Autodesk Fusion 360 part; units mm, degrees
note: some values were not read from the file. Set by a fixed rule: which sketch regions a step uses.
(part 2 of 2)
sketch "Sketch3" plane through (0, 0, 0) normal (0, 0, -1) x (1, 0, 0)
  line L0 (-14.5833, -10.5) -> (-14.5833, -10.5839)
  arc A0 (-8, -23) -> (-14.5833, -10.5839) centre (-23, -23) ccw
  line L1 (-8, -23) -> (-8, -42.8293)
  arc A1 (-10.0769, -45.2933) -> (-8, -42.8293) centre (-10.5, -42.8293) ccw
  arc A2 (-10.0769, -45.2933) -> (-10.4615, -55.0673) centre (-9.2308, -50.2212) ccw
  arc A3 (-10.4615, -55.0673) -> (10.4615, -55.0673) centre (0, -13.875) ccw
  arc A4 (10.4615, -55.0673) -> (10.0769, -45.2933) centre (9.2308, -50.2212) ccw
  arc A5 (8, -42.8293) -> (10.0769, -45.2933) centre (10.5, -42.8293) ccw
  line L2 (8, -42.8293) -> (8, -23)
  arc A6 (14.5833, -10.5839) -> (8, -23) centre (23, -23) ccw
  line L3 (14.5833, -10.5839) -> (14.5833, -10.5)
  line L4 (14.5833, -10.5) -> (14.7084, -10.5)
  arc A7 (23, -8) -> (14.7084, -10.5) centre (23, -23) ccw
  line L5 (23, -8) -> (42.8293, -8)
  arc A8 (45.2933, -10.0769) -> (42.8293, -8) centre (42.8293, -10.5) ccw
  arc A9 (45.2933, -10.0769) -> (55.0673, -10.4615) centre (50.2212, -9.2308) ccw
  arc A10 (55.0673, -10.4615) -> (55.0673, 10.4615) centre (13.875, 0) ccw
  arc A11 (55.0673, 10.4615) -> (45.2933, 10.0769) centre (50.2212, 9.2308) ccw
  arc A12 (42.8293, 8) -> (45.2933, 10.0769) centre (42.8293, 10.5) ccw
  line L6 (42.8293, 8) -> (23, 8)
  arc A13 (8, 23) -> (23, 8) centre (23, 23) ccw
  line L7 (8, 23) -> (8, 42.8293)
  arc A14 (10.0769, 45.2933) -> (8, 42.8293) centre (10.5, 42.8293) ccw
  arc A15 (10.0769, 45.2933) -> (10.4615, 55.0673) centre (9.2308, 50.2212) ccw
  arc A16 (10.4615, 55.0673) -> (-10.4615, 55.0673) centre (0, 13.875) ccw
  arc A17 (-10.4615, 55.0673) -> (-10.0769, 45.2933) centre (-9.2308, 50.2212) ccw
  arc A18 (-8, 42.8293) -> (-10.0769, 45.2933) centre (-10.5, 42.8293) ccw
  line L8 (-8, 42.8293) -> (-8, 23)
  arc A19 (-23, 8) -> (-8, 23) centre (-23, 23) ccw
  line L9 (-23, 8) -> (-42.8293, 8)
  arc A20 (-45.2933, 10.0769) -> (-42.8293, 8) centre (-42.8293, 10.5) ccw
  arc A21 (-45.2933, 10.0769) -> (-55.0673, 10.4615) centre (-50.2212, 9.2308) ccw
  arc A22 (-55.0673, 10.4615) -> (-55.0673, -10.4615) centre (-13.875, 0) ccw
  arc A23 (-55.0673, -10.4615) -> (-45.2933, -10.0769) centre (-50.2212, -9.2308) ccw
  arc A24 (-42.8293, -8) -> (-45.2933, -10.0769) centre (-42.8293, -10.5) ccw
  line L10 (-42.8293, -8) -> (-23, -8)
  arc A25 (-14.7084, -10.5) -> (-23, -8) centre (-23, -23) ccw
  line L11 (-14.7084, -10.5) -> (-14.5833, -10.5)
  line L12 (-8.3333, -9.25) -> (-8.3333, -5.25)
  line L13 (-8.3333, -5.25) -> (-10.3333, -5.25)
  line L14 (-10.3333, -5.25) -> (-10.3333, -3.25)
  line L15 (-10.3333, -3.25) -> (-8.3333, -3.25)
  line L16 (-8.3333, -3.25) -> (-8.3333, -1.25)
  line L17 (-8.3333, -1.25) -> (-6.3333, -1.25)
  line L18 (-6.3333, -1.25) -> (-6.3333, -3.25)
  line L19 (-6.3333, -3.25) -> (-4.3333, -3.25)
  line L20 (-4.3333, -3.25) -> (-4.3333, -5.25)
  line L21 (-4.3333, -5.25) -> (-6.3333, -5.25)
  line L22 (-6.3333, -5.25) -> (-6.3333, -9.25)
  line L23 (-6.3333, -9.25) -> (-8.3333, -9.25)
  line L24 (-1.25, -10.5) -> (-1.25, -8)
  line L25 (-1.25, -8) -> (1.25, -8)
  line L26 (1.25, -8) -> (1.25, -10.5)
  line L27 (1.25, -10.5) -> (3.75, -10.5)
  line L28 (3.75, -10.5) -> (3.75, -13)
  line L29 (3.75, -13) -> (1.25, -13)
  line L30 (1.25, -13) -> (1.25, -18)
  line L31 (1.25, -18) -> (-1.25, -18)
  line L32 (-1.25, -18) -> (-1.25, -13)
  line L33 (-1.25, -13) -> (-3.75, -13)
  line L34 (-3.75, -13) -> (-3.75, -10.5)
  line L35 (-3.75, -10.5) -> (-1.25, -10.5)
  line L36 (-41.25, 2.5) -> (-41.25, 5)
  line L37 (-41.25, 5) -> (-38.75, 5)
  line L38 (-38.75, 5) -> (-38.75, 2.5)
  line L39 (-38.75, 2.5) -> (-36.25, 2.5)
  line L40 (-36.25, 2.5) -> (-36.25, 0)
  line L41 (-36.25, 0) -> (-38.75, 0)
  line L42 (-38.75, 0) -> (-38.75, -5)
  line L43 (-38.75, -5) -> (-41.25, -5)
  line L44 (-41.25, -5) -> (-41.25, 0)
  line L45 (-41.25, 0) -> (-43.75, 0)
  line L46 (-43.75, 0) -> (-43.75, 2.5)
  line L47 (-43.75, 2.5) -> (-41.25, 2.5)
  line L48 (12.0833, 2.5) -> (12.0833, 5)
  line L49 (12.0833, 5) -> (14.5833, 5)
  line L50 (14.5833, 5) -> (14.5833, 2.5)
  line L51 (14.5833, 2.5) -> (17.0833, 2.5)
  line L52 (17.0833, 2.5) -> (17.0833, 0)
  line L53 (17.0833, 0) -> (14.5833, 0)
  line L54 (14.5833, 0) -> (14.5833, -5)
  line L55 (14.5833, -5) -> (12.0833, -5)
  line L56 (12.0833, -5) -> (12.0833, 0)
  line L57 (12.0833, 0) -> (9.5833, 0)
  line L58 (9.5833, 0) -> (9.5833, 2.5)
  line L59 (9.5833, 2.5) -> (12.0833, 2.5)
  line L60 (25.4167, 2.5) -> (25.4167, 5)
  line L61 (25.4167, 5) -> (27.9167, 5)
  line L62 (27.9167, 5) -> (27.9167, 2.5)
  line L63 (27.9167, 2.5) -> (30.4167, 2.5)
  line L64 (30.4167, 2.5) -> (30.4167, 0)
  line L65 (30.4167, 0) -> (27.9167, 0)
  line L66 (27.9167, 0) -> (27.9167, -5)
  line L67 (27.9167, -5) -> (25.4167, -5)
  line L68 (25.4167, -5) -> (25.4167, 0)
  line L69 (25.4167, 0) -> (22.9167, 0)
  line L70 (22.9167, 0) -> (22.9167, 2.5)
  line L71 (22.9167, 2.5) -> (25.4167, 2.5)
  line L72 (-14.5833, 2.5) -> (-14.5833, 5)
  line L73 (-14.5833, 5) -> (-12.0833, 5)
  line L74 (-12.0833, 5) -> (-12.0833, 2.5)
  line L75 (-12.0833, 2.5) -> (-9.5833, 2.5)
  line L76 (-9.5833, 2.5) -> (-9.5833, 0)
  line L77 (-9.5833, 0) -> (-12.0833, 0)
  line L78 (-12.0833, 0) -> (-12.0833, -5)
  line L79 (-12.0833, -5) -> (-14.5833, -5)
  line L80 (-14.5833, -5) -> (-14.5833, 0)
  line L81 (-14.5833, 0) -> (-17.0833, 0)
  line L82 (-17.0833, 0) -> (-17.0833, 2.5)
  line L83 (-17.0833, 2.5) -> (-14.5833, 2.5)
  line L84 (-1.25, 41.5) -> (-1.25, 44)
  line L85 (-1.25, 44) -> (1.25, 44)
  line L86 (1.25, 44) -> (1.25, 41.5)
  line L87 (1.25, 41.5) -> (3.75, 41.5)
  line L88 (3.75, 41.5) -> (3.75, 39)
  line L89 (3.75, 39) -> (1.25, 39)
  line L90 (1.25, 39) -> (1.25, 34)
  line L91 (1.25, 34) -> (-1.25, 34)
  line L92 (-1.25, 34) -> (-1.25, 39)
  line L93 (-1.25, 39) -> (-3.75, 39)
  line L94 (-3.75, 39) -> (-3.75, 41.5)
  line L95 (-3.75, 41.5) -> (-1.25, 41.5)
  line L96 (-1.25, -23.5) -> (-1.25, -21)
  line L97 (-1.25, -21) -> (1.25, -21)
  line L98 (1.25, -21) -> (1.25, -23.5)
  line L99 (1.25, -23.5) -> (3.75, -23.5)
  line L100 (3.75, -23.5) -> (3.75, -26)
  line L101 (3.75, -26) -> (1.25, -26)
  line L102 (1.25, -26) -> (1.25, -31)
  line L103 (1.25, -31) -> (-1.25, -31)
  line L104 (-1.25, -31) -> (-1.25, -26)
  line L105 (-1.25, -26) -> (-3.75, -26)
  line L106 (-3.75, -26) -> (-3.75, -23.5)
  line L107 (-3.75, -23.5) -> (-1.25, -23.5)
  line L108 (-3.75, 2.5) -> (-1.25, 2.5)
  line L109 (-1.25, 2.5) -> (-1.25, 5)
  line L110 (-1.25, 5) -> (1.25, 5)
  line L111 (1.25, 5) -> (1.25, 2.5)
  line L112 (1.25, 2.5) -> (3.75, 2.5)
  line L113 (3.75, 2.5) -> (3.75, 0)
  line L114 (3.75, 0) -> (1.25, 0)
  line L115 (1.25, 0) -> (1.25, -5)
  line L116 (1.25, -5) -> (-1.25, -5)
  line L117 (-1.25, -5) -> (-1.25, 0)
  line L118 (-1.25, 0) -> (-3.75, 0)
  line L119 (-3.75, 0) -> (-3.75, 2.5)
  line L120 (-1.25, 28.5) -> (-1.25, 31)
  line L121 (-1.25, 31) -> (1.25, 31)
  line L122 (1.25, 31) -> (1.25, 28.5)
  line L123 (1.25, 28.5) -> (3.75, 28.5)
  line L124 (3.75, 28.5) -> (3.75, 26)
  line L125 (3.75, 26) -> (1.25, 26)
  line L126 (1.25, 26) -> (1.25, 21)
  line L127 (1.25, 21) -> (-1.25, 21)
  line L128 (-1.25, 21) -> (-1.25, 26)
  line L129 (-1.25, 26) -> (-3.75, 26)
  line L130 (-3.75, 26) -> (-3.75, 28.5)
  line L131 (-3.75, 28.5) -> (-1.25, 28.5)
  line L132 (-27.9167, 2.5) -> (-27.9167, 5)
  line L133 (-27.9167, 5) -> (-25.4167, 5)
  line L134 (-25.4167, 5) -> (-25.4167, 2.5)
  line L135 (-25.4167, 2.5) -> (-22.9167, 2.5)
  line L136 (-22.9167, 2.5) -> (-22.9167, 0)
  line L137 (-22.9167, 0) -> (-25.4167, 0)
  line L138 (-25.4167, 0) -> (-25.4167, -5)
  line L139 (-25.4167, -5) -> (-27.9167, -5)
  line L140 (-27.9167, -5) -> (-27.9167, 0)
  line L141 (-27.9167, 0) -> (-30.4167, 0)
  line L142 (-30.4167, 0) -> (-30.4167, 2.5)
  line L143 (-30.4167, 2.5) -> (-27.9167, 2.5)
  line L144 (3.75, 9.75) -> (5.6667, 9.75)
  line L145 (5.6667, 9.75) -> (5.6667, 11.75)
  line L146 (5.6667, 11.75) -> (7.6667, 11.75)
  line L147 (7.6667, 11.75) -> (7.6667, 9.75)
  line L148 (7.6667, 9.75) -> (9.6667, 9.75)
  line L149 (9.6667, 9.75) -> (9.6667, 7.75)
  line L150 (9.6667, 7.75) -> (7.6667, 7.75)
  line L151 (7.6667, 7.75) -> (7.6667, 3.75)
  line L152 (7.6667, 3.75) -> (5.6667, 3.75)
  line L153 (5.6667, 3.75) -> (5.6667, 7.75)
  line L154 (5.6667, 7.75) -> (3.75, 7.75)
  line L155 (3.75, 7.75) -> (3.75, 9.75)
  line L156 (5.6667, -9.25) -> (5.6667, -5.25)
  line L157 (5.6667, -5.25) -> (3.6667, -5.25)
  line L158 (3.6667, -5.25) -> (3.6667, -3.25)
  line L159 (3.6667, -3.25) -> (5.6667, -3.25)
  line L160 (5.6667, -3.25) -> (5.6667, -1.25)
  line L161 (5.6667, -1.25) -> (7.6667, -1.25)
  line L162 (7.6667, -1.25) -> (7.6667, -3.25)
  line L163 (7.6667, -3.25) -> (9.6667, -3.25)
  line L164 (9.6667, -3.25) -> (9.6667, -5.25)
  line L165 (9.6667, -5.25) -> (7.6667, -5.25)
  line L166 (7.6667, -5.25) -> (7.6667, -9.25)
  line L167 (7.6667, -9.25) -> (5.6667, -9.25)
  line L168 (38.75, 2.5) -> (38.75, 5)
  line L169 (38.75, 5) -> (41.25, 5)
  line L170 (41.25, 5) -> (41.25, 2.5)
  line L171 (41.25, 2.5) -> (43.75, 2.5)
  line L172 (43.75, 2.5) -> (43.75, 0)
  line L173 (43.75, 0) -> (41.25, 0)
  line L174 (41.25, 0) -> (41.25, -5)
  line L175 (41.25, -5) -> (38.75, -5)
  line L176 (38.75, -5) -> (38.75, 0)
  line L177 (38.75, 0) -> (36.25, 0)
  line L178 (36.25, 0) -> (36.25, 2.5)
  line L179 (36.25, 2.5) -> (38.75, 2.5)
  line L180 (-1.25, -36.5) -> (-1.25, -34)
  line L181 (-1.25, -34) -> (1.25, -34)
  line L182 (1.25, -34) -> (1.25, -36.5)
  line L183 (1.25, -36.5) -> (3.75, -36.5)
  line L184 (3.75, -36.5) -> (3.75, -39)
  line L185 (3.75, -39) -> (1.25, -39)
  line L186 (1.25, -39) -> (1.25, -44)
  line L187 (1.25, -44) -> (-1.25, -44)
  line L188 (-1.25, -44) -> (-1.25, -39)
  line L189 (-1.25, -39) -> (-3.75, -39)
  line L190 (-3.75, -39) -> (-3.75, -36.5)
  line L191 (-3.75, -36.5) -> (-1.25, -36.5)
  line L192 (-1.25, 15.5) -> (-1.25, 18)
  line L193 (-1.25, 18) -> (1.25, 18)
  line L194 (1.25, 18) -> (1.25, 15.5)
  line L195 (1.25, 15.5) -> (3.75, 15.5)
  line L196 (3.75, 15.5) -> (3.75, 13)
  line L197 (3.75, 13) -> (1.25, 13)
  line L198 (1.25, 13) -> (1.25, 8)
  line L199 (1.25, 8) -> (-1.25, 8)
  line L200 (-1.25, 8) -> (-1.25, 13)
  line L201 (-1.25, 13) -> (-3.75, 13)
  line L202 (-3.75, 13) -> (-3.75, 15.5)
  line L203 (-3.75, 15.5) -> (-1.25, 15.5)
  line L204 (-8.3333, 3.75) -> (-8.3333, 7.75)
  line L205 (-8.3333, 7.75) -> (-10.3333, 7.75)
  line L206 (-10.3333, 7.75) -> (-10.3333, 9.75)
  line L207 (-10.3333, 9.75) -> (-8.3333, 9.75)
  line L208 (-8.3333, 9.75) -> (-8.3333, 11.75)
  line L209 (-8.3333, 11.75) -> (-6.3333, 11.75)
  line L210 (-6.3333, 11.75) -> (-6.3333, 9.75)
  line L211 (-6.3333, 9.75) -> (-4.3333, 9.75)
  line L212 (-4.3333, 9.75) -> (-4.3333, 7.75)
  line L213 (-4.3333, 7.75) -> (-6.3333, 7.75)
  line L214 (-6.3333, 7.75) -> (-6.3333, 3.75)
  line L215 (-6.3333, 3.75) -> (-8.3333, 3.75)
  circle A26 centre (0, 51.375) radius 2.5
  circle A27 centre (-51.375, 0) radius 2.5
  circle A28 centre (51.375, 0) radius 2.5
  circle A29 centre (0, -51.375) radius 2.5
  circle A30 centre (-51.375, 0) radius 4.25
  circle A31 centre (0, -51.375) radius 4.25
  circle A32 centre (51.375, 0) radius 4.25
  circle A33 centre (0, 51.375) radius 4.25
  dimension "d51" = 8.5
  dimension "d53" = 360
  constraint concentric A27 A30
  measures "d51" diameter of A30
extrude "Extrude4" cut sketch "Sketch3" against normal blind 3 contours A30 | A31 | A32 | A33
equation "d17 = 4 mm + 5 mm"
equation "d26 = d25 / 4"
equation "d27 = d26 * 2"
equation "d28 = d25 * 2"
